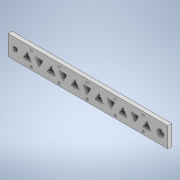
# Autodesk Inventor part: arm_plate_btw_support_bicep
Saved by Autodesk Inventor 2022 (Build 260153000, 153)
## iProperties
Created: 2022-01-24
Part Number: arm_plate_btw_support_bicep
Material: Generic
Document SubType Name: Modeling
Designer: pauly
Density: 1 g/cm^3
Appearance: Default
Author: pauly
Autodesk Inventor part; units mm, degrees
ref_plane "YZ Plane" through (0, 0, 0) normal (1, 0, 0) x (0, 1, 0)
ref_plane "XZ Plane" through (0, 0, 0) normal (0, 1, 0) x (-1, 0, 0)
ref_plane "XY Plane" through (0, 0, 0) normal (0, 0, 1) x (1, 0, 0)
sketch "Sketch1" plane through (0, 0, 0) normal (0, 0, 1) x (1, 0, 0)
  line L0 (0, 0) -> (508, 0)
  line L1 (508, 0) -> (508, 63.5)
  line L2 (508, 63.5) -> (0, 63.5)
  line L3 (0, 63.5) -> (0, 0)
  circle A0 centre (484.886, 31.75) radius 10.9982
  circle A1 centre (73.914, 53.3905) radius 3.175
  circle A2 centre (162.9664, 53.3905) radius 3.175
  circle A3 centre (252.0188, 53.3868) radius 3.175
  circle A4 centre (341.0712, 53.3868) radius 3.175
  circle A5 centre (430.1236, 53.3868) radius 3.175
  circle A6 centre (73.914, 8.9405) radius 3.175
  circle A7 centre (162.9664, 8.9368) radius 3.175
  circle A8 centre (252.0188, 8.9368) radius 3.175
  circle A9 centre (341.0712, 8.9368) radius 3.175
  circle A10 centre (430.1236, 8.9368) radius 3.175
  line L4 (61.214, 43.0781) -> (73.5873, 21.6469)
  line L5 (48.8407, 21.6469) -> (61.214, 43.0781)
  line L6 (137.414, 43.0781) -> (149.7873, 21.6469)
  line L7 (149.7873, 21.6469) -> (125.0407, 21.6469)
  line L8 (125.0407, 21.6469) -> (137.414, 43.0781)
  line L9 (99.314, 21.6469) -> (86.9407, 43.0781)
  line L10 (86.9407, 43.0781) -> (111.6873, 43.0781)
  line L11 (111.6873, 43.0781) -> (99.314, 21.6469)
  line L12 (26.7802, 38.1) -> (30.4463, 31.75)
  line L13 (30.4463, 31.75) -> (26.7681, 25.4)
  line L14 (26.7681, 25.4) -> (19.4478, 25.4)
  line L15 (19.4478, 25.4) -> (15.7817, 31.75)
  line L16 (15.7817, 31.75) -> (19.4478, 38.1)
  line L17 (19.4478, 38.1) -> (26.7802, 38.1)
  line L18 (48.8407, 21.6469) -> (73.5873, 21.6469)
  line L19 (289.4838, 43.0781) -> (301.8571, 21.6469)
  line L20 (301.8571, 21.6469) -> (277.1105, 21.6469)
  line L21 (277.1105, 21.6469) -> (289.4838, 43.0781)
  line L22 (263.7571, 43.0781) -> (251.3838, 21.6469)
  line L23 (251.3838, 21.6469) -> (239.0105, 43.0781)
  line L24 (239.0105, 43.0781) -> (263.7571, 43.0781)
  line L25 (213.2838, 43.0781) -> (225.6571, 21.6469)
  line L26 (200.9105, 21.6469) -> (225.6571, 21.6469)
  line L27 (200.9105, 21.6469) -> (213.2838, 43.0781)
  line L28 (441.5536, 43.0781) -> (453.9269, 21.6469)
  line L29 (453.9269, 21.6469) -> (429.1803, 21.6469)
  line L30 (429.1803, 21.6469) -> (441.5536, 43.0781)
  line L31 (415.8269, 43.0781) -> (403.4536, 21.6469)
  line L32 (403.4536, 21.6469) -> (391.0803, 43.0781)
  line L33 (391.0803, 43.0781) -> (415.8269, 43.0781)
  line L34 (365.3536, 43.0781) -> (377.7269, 21.6469)
  line L35 (352.9803, 21.6469) -> (377.7269, 21.6469)
  line L36 (352.9803, 21.6469) -> (365.3536, 43.0781)
  line L37 (175.5175, 21.6469) -> (163.1442, 43.0781)
  line L38 (163.1442, 43.0781) -> (187.8909, 43.0781)
  line L39 (187.8909, 43.0781) -> (175.5175, 21.6469)
  line L40 (339.9607, 43.0781) -> (327.5873, 21.6469)
  line L41 (327.5873, 21.6469) -> (315.214, 43.0781)
  line L42 (315.214, 43.0781) -> (339.9607, 43.0781)
  point P0 (135.1884, 47.8306)
  point P1 (135.1884, 33.5431)
  point P2 (23.114, 19.05)
  point P3 (23.114, 25.4)
  point P4 (287.2582, 33.5431)
  point P5 (439.328, 33.5431)
  dimension "d18" = 44.45
  dimension "d36" = 56.5658
  dimension "d69" = 126.3396
  dimension "d72" = 25.4
  dimension "d0" = 508
  dimension "d1" = 63.5
  dimension "d3" = 21.9964
  dimension "d12" = 6.35
  dimension "d15" = 89.0524
  dimension "d44" = 6.35
  dimension "d66" = 100.9467
  dimension "d91" = 22.0726
  dimension "d97" = 152.0698
  dimension "d102" = 51.1231
  constraints: 86 end point, 11 centre point, 5 horizontal, 2 parallel, 1 collinear, 1 perpendicular, 1 vertical, 40 other
  measures "d0" distance of L2.end L1.end
  measures "d1" distance of L1.end L0.end
  measures "d3" diameter of A0
  measures "d12" diameter of A1
  measures "d15" distance of A1.centre A2.centre
  measures "d44" diameter of A2
  measures "d66" distance of L6.end L5.start
  measures "d91" horizontal distance of L13.end L5.start
  measures "d97" distance of L6.end L19.end
  measures "d102" distance of L26.start L6.end
extrude "Extrusion1" add sketch "Sketch1" along normal blind 12.7 contours L3 L2 L1 L0 | L4 L18 L5 | L12 L13 L14 L15 L16 L17 | L19 L20 L21 | L22 L23 L24 | L25 L26 L27 | L28 L29 L30 | L31 L32 L33 | L34 L35 L36 | L37 L38 L39 | L40 L41 L42
extrude "Extrusion2" cut sketch "Sketch1" along normal blind 25.4 contours L12 L13 L14 L15 L16 L17
extrude "Extrusion4" cut sketch "Sketch1" along normal blind 12.7 contours L4 L18 L5
extrude "Extrusion5" cut sketch "Sketch1" along normal blind 12.7 contours L19 L20 L21 | L22 L23 L24 | L25 L26 L27 | L28 L29 L30 | L31 L32 L33 | L34 L35 L36 | L37 L38 L39 | L40 L41 L42
body "Solid1"
